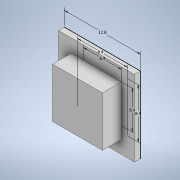
# Autodesk Inventor part: reset button cover
Saved by Autodesk Inventor 2022 (Build 260153000, 153)
## iProperties
Created: 2022-06-09
Part Number: reset button cover
Material: Generic
Document SubType Name: Modeling
Designer: alecw
Density: 1 g/cm^3
Appearance: Default
Author: alecw
Autodesk Inventor part; units mm, degrees
ref_plane "YZ Plane" through (0, 0, 0) normal (1, 0, 0) x (0, 1, 0)
ref_plane "XZ Plane" through (0, 0, 0) normal (0, 1, 0) x (-1, 0, 0)
ref_plane "XY Plane" through (0, 0, 0) normal (0, 0, 1) x (1, 0, 0)
sketch "Sketch1" plane through (0, 0, 0) normal (0, 0, 1) x (1, 0, 0)
  line L0 (-3.2, -3.2) -> (3.2, -3.2)
  line L1 (3.2, -3.2) -> (3.2, 3.2)
  line L2 (3.2, 3.2) -> (-3.2, 3.2)
  line L3 (-3.2, 3.2) -> (-3.2, -3.2)
  line L4 (-3.2, -3.2) -> (3.2, 3.2) construction
  line L5 (3.2, -3.2) -> (-3.2, 3.2) construction
  line L6 (-4.2, 4.2) -> (4.2, 4.2)
  line L7 (4.2, 4.2) -> (4.2, -4.2)
  line L8 (4.2, -4.2) -> (-4.2, -4.2)
  line L9 (-4.2, -4.2) -> (-4.2, 4.2)
  line L10 (-4.2, 4.2) -> (4.2, -4.2) construction
  line L11 (4.2, 4.2) -> (-4.2, -4.2) construction
  line L12 (6.4, -6.4) -> (-6.4, -6.4)
  line L13 (-6.4, -6.4) -> (-6.4, 6.4)
  line L14 (-6.4, 6.4) -> (6.4, 6.4)
  line L15 (6.4, 6.4) -> (6.4, -6.4)
  line L16 (6.4, -6.4) -> (-6.4, 6.4) construction
  line L17 (-6.4, -6.4) -> (6.4, 6.4) construction
  point P0 (0, 0)
  dimension "d0" = 6.4
  dimension "d1" = 6.4
  dimension "d2" = 8.4
  dimension "d3" = 8.4
  dimension "d4" = 12.8
  constraints: 36 end point, 6 midpoint, 6 parallel, 3 horizontal, 3 perpendicular, 1 point on line
  measures "d0" distance of L2.end L1.end
  measures "d1" distance of L1.end L0.end
  measures "d2" distance of L7.end L8.end
  measures "d3" distance of L6.end L7.end
  measures "d4" distance of L13.end L14.end
extrude "Extrusion1" add sketch "Sketch1" along normal blind 1 contours L6 L7 L8 L9 | L12 L13 L14 L15
extrude "Extrusion2" add sketch "Sketch1" along normal blind 3.2 from surface at 1 contours L6 L7 L8 L9
extrude "Extrusion3" add sketch "Sketch1" against normal blind 2 from surface at 4.2 contours L3 L2 L1 L0 | L6 L7 L8 L9
body "Solid1"
